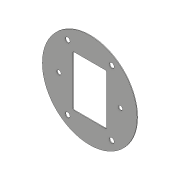
# Autodesk Inventor part: fanFlange
Saved by Autodesk Inventor 2017 (Build 210142000, 142)
## iProperties
Created: 2017-05-16
Part Number: fanFlange
Material: Generic
Document SubType Name: Sheet Metal
Designer: krosie
Density: 1 g/cm^3
Sheet Metal Rule: Default_mm
Appearance: Default
Author: krosie
Autodesk Inventor part; units mm, degrees
ref_plane "YZ Plane" through (0, 0, 0) normal (1, 0, 0) x (0, 1, 0)
ref_plane "XZ Plane" through (0, 0, 0) normal (0, 1, 0) x (-1, 0, 0)
ref_plane "XY Plane" through (0, 0, 0) normal (0, 0, 1) x (1, 0, 0)
sketch "Sketch1" plane through (0, 0, 0) normal (0, 1, 0) x (-1, 0, 0)
  line L0 (-26, 39) -> (26, 39)
  line L1 (26, 39) -> (26, -39)
  line L2 (26, -39) -> (-26, -39)
  line L3 (-26, -39) -> (-26, 39)
  line L4 (-26, 39) -> (26, -39) construction
  line L5 (26, 39) -> (-26, -39) construction
  line L6 (-42, 57.5) -> (42, 57.5)
  line L7 (42, 57.5) -> (42, -57.5)
  line L8 (42, -57.5) -> (-42, -57.5)
  line L9 (-42, -57.5) -> (-42, 57.5)
  line L10 (-42, 57.5) -> (42, -57.5) construction
  line L11 (42, 57.5) -> (-42, -57.5) construction
  line L12 (-34, 50) -> (34, 50) construction
  line L13 (34, 50) -> (34, -50) construction
  line L14 (34, -50) -> (-34, -50) construction
  line L15 (-34, -50) -> (-34, 50) construction
  line L16 (-34, 50) -> (34, -50) construction
  line L17 (34, 50) -> (-34, -50) construction
  circle A0 centre (34, 50) radius 3.75
  circle A1 centre (34, -50) radius 3.75
  circle A2 centre (-34, -50) radius 3.75
  circle A3 centre (-34, 50) radius 3.75
  point P0 (0, 0)
  dimension "d0" = 52
  dimension "d1" = 78
  dimension "d2" = 84
  dimension "d3" = 115
  dimension "d4" = 68
  dimension "d5" = 100
  dimension "d6" = 7.5
  dimension "d7" = 7.5
  dimension "d8" = 7.5
  dimension "d9" = 7.5
  measures "d0" distance of L1.end L2.end
  measures "d1" distance of L0.end L1.end
  measures "d2" distance of L7.end L8.end
  measures "d3" distance of L6.end L7.end
  measures "d4" distance of L13.end L14.end
  measures "d5" distance of L12.end L13.end
  measures "d6" diameter of A0
  measures "d7" diameter of A1
  measures "d8" diameter of A2
  measures "d9" diameter of A3
extrude "Plate1" add sketch "Sketch1" along normal blind 1
sketch "Sketch2" plane through (0, 0, 0) normal (0, -1, 0) x (1, 0, 0)
  circle A0 centre (0, 0) radius 73
  circle A1 centre (-34, 50) radius 3.75
  circle A2 centre (34, 50) radius 3.75
  circle A3 centre (34, -50) radius 3.75
  circle A4 centre (-34, -50) radius 3.75
  line L0 (-26, -39) -> (-26, 39)
  line L1 (-26, 39) -> (26, 39)
  line L2 (26, 39) -> (26, -39)
  line L3 (26, -39) -> (-26, -39)
  dimension "d18" = 146
  measures "d18" diameter of A0
sheet face with bend "Face3" sketch "Sketch2" thickness 1 toward (0, 1, 0) bend radius 1 relief straight relief width 1 relief depth 0.5
bend "Bend2"
sketch "Sketch3" plane through (0, 0, 0) normal (0, -1, 0) x (1, 0, 0)
  circle A0 centre (0, 0) radius 52.7 construction
  circle A1 centre (-47.35, 0) radius 3.25
  circle A2 centre (47.35, 0) radius 3.25
  line L0 (-52.7, 0) -> (-42, 0) construction
  line L1 (42, 0) -> (52.7, 0) construction
  dimension "d24" = 105.4
  dimension "d26" = 6.5
  dimension "d27" = 6.5
  constraints: 4 end point, 3 centre point, 2 horizontal, 2 midpoint, 2 point on circle, 1 coincident
  measures "d24" diameter of A0
  measures "d26" diameter of A1
  measures "d27" diameter of A2
extrude "Cut1" cut sketch "Sketch3" against normal blind 1
fillet "Fillet1" radius 2 4 edges at (-26, 0.5, 39) (26, 0.5, 39) (26, 0.5, -39) (-26, 0.5, -39)
equation "\"d28\" = Thickness"
equation "\"d19\" = BendRadius"
equation "\"d20\" = BendReliefWidth"
equation "\"d22\" = MinimumRemnant"
equation "\"d21\" = BendReliefDepth"
equation "\"d23\" = BendRadius"
equation "\"BendRadius\" = Thickness"
equation "\"BendReliefWidth\" = Thickness"
equation "\"BendReliefDepth\" = 0.5 * Thickness"
equation "\"CornerReliefSize\" = 4 * Thickness"
equation "\"MinimumRemnant\" = 2 * Thickness"
equation "\"TransitionRadius\" = BendRadius"
equation "\"JacobiRadiusSize\" = BendRadius"
equation "\"GapSize\" = Thickness"
equation "\"d10\" = BendRadius"
equation "\"Thickness\" = 1"
body "Solid1"
